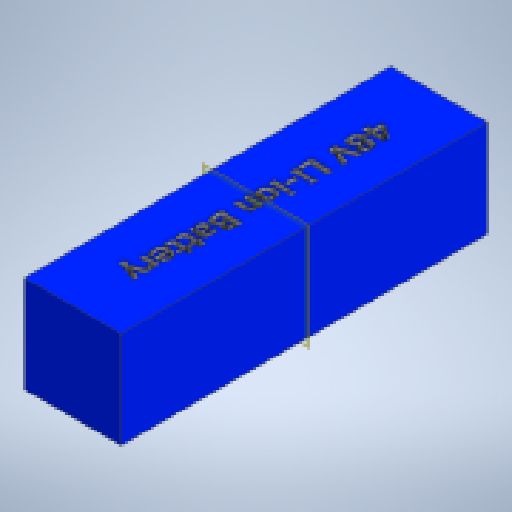
# Autodesk Inventor part: Battery
Saved by Autodesk Inventor 2026.2 (Build 302298010, 298A)
## iProperties
Created: 2026-03-27
Part Number: Battery
Material: Generic
Document SubType Name: Modeling
Designer: chanh
Density: 1 g/cm^3
Appearance: Default
Author: chanh
Autodesk Inventor part; units mm, degrees
ref_plane "YZ Plane" through (0, 0, 0) normal (1, 0, 0) x (0, 1, 0)
ref_plane "XZ Plane" through (0, 0, 0) normal (0, 1, 0) x (-1, 0, 0)
ref_plane "XY Plane" through (0, 0, 0) normal (0, 0, 1) x (1, 0, 0)
sketch "Sketch1" plane through (0, 0, 0) normal (0, 0, 1) x (1, 0, 0)
  line L0 (-35, -35) -> (35, -35)
  line L1 (35, -35) -> (35, 35)
  line L2 (35, 35) -> (-35, 35)
  line L3 (-35, 35) -> (-35, -35)
  line L4 (-35, -35) -> (35, 35) construction
  line L5 (35, -35) -> (-35, 35) construction
  point P0 (0, 0)
  dimension "d0" = 70
  dimension "d1" = 70
  constraints: 12 end point, 2 midpoint, 2 parallel, 1 horizontal, 1 perpendicular
  measures "d0" distance of L1.end L2.end
  measures "d1" distance of L0.end L1.end
extrude "Extrusion1" add sketch "Sketch1" along normal blind 265
sketch "Sketch2" plane through (-35, 35, 0) normal (0, 1, 0) x (1, 0, 0)
  line L0 (44.9615, -38.8119) -> (44.9615, -229.4187) construction
  line L1 (44.9615, -229.4187) -> (21.1166, -229.4187) construction
  line L2 (21.1166, -229.4187) -> (21.1166, -38.8119) construction
  line L3 (21.1166, -38.8119) -> (44.9615, -38.8119) construction
  line L4 (32.7816, -51.5388) -> (32.7816, -49.5088)
  line L5 (32.7816, -49.5088) -> (29.2443, -49.5088)
  line L6 (29.2443, -49.5088) -> (29.2443, -45.8743)
  line L7 (29.2443, -45.8743) -> (32.7816, -45.8743)
  line L8 (32.7816, -45.8743) -> (32.7816, -39.2616)
  line L9 (32.7816, -39.2616) -> (35.5774, -39.2616)
  line L10 (35.5774, -39.2616) -> (44.2808, -45.7527)
  line L11 (44.2808, -45.7527) -> (44.2808, -49.5088)
  line L12 (44.2808, -49.5088) -> (35.4801, -49.5088)
  line L13 (35.4801, -49.5088) -> (35.4801, -51.5388)
  line L14 (35.4801, -51.5388) -> (32.7816, -51.5388)
  line L15 (35.4801, -45.8743) -> (40.5855, -45.8743)
  line L16 (40.5855, -45.8743) -> (35.4801, -42.0696)
  line L17 (35.4801, -42.0696) -> (35.4801, -45.8743)
  spline S0 degree 2 poles (33.4502, -64.4602) (32.4899, -64.4602) (30.8245, -63.6579) (30.2168, -62.8921) knots 0 0 0 1 2 2 2
  spline S1 degree 2 poles (30.2168, -62.8921) (29.609, -62.1263) (28.9283, -59.9261) (28.9283, -58.5039) knots 0 0 0 1 2 2 2
  spline S2 degree 2 poles (28.9283, -58.5039) (28.9283, -56.9845) (29.6211, -54.7114) (30.2168, -53.9821) knots 0 0 0 1 2 2 2
  spline S3 degree 2 poles (30.2168, -53.9821) (30.8124, -53.2649) (32.4291, -52.5842) (33.3286, -52.5842) knots 0 0 0 1 2 2 2
  spline S4 degree 2 poles (33.3286, -52.5842) (34.6171, -52.5842) (36.331, -54.0064) (36.9023, -55.3556) knots 0 0 0 1 2 2 2
  line L18 (36.9023, -55.3556) -> (36.9631, -55.3556)
  spline S5 degree 2 poles (36.9631, -55.3556) (37.6074, -54.0307) (39.4429, -52.9853) (40.5733, -52.9853) knots 0 0 0 1 2 2 2
  spline S6 degree 2 poles (40.5733, -52.9853) (41.3999, -52.9853) (42.8464, -53.7146) (43.4177, -54.4318) knots 0 0 0 1 2 2 2
  spline S7 degree 2 poles (43.4177, -54.4318) (43.9647, -55.1247) (44.6211, -57.2276) (44.6211, -58.5404) knots 0 0 0 1 2 2 2
  spline S8 degree 2 poles (44.6211, -58.5404) (44.6211, -59.9261) (44.0255, -61.9926) (43.5393, -62.6612) knots 0 0 0 1 2 2 2
  spline S9 degree 2 poles (43.5393, -62.6612) (43.0531, -63.3419) (41.643, -64.0712) (40.8286, -64.0712) knots 0 0 0 1 2 2 2
  spline S10 degree 2 poles (40.8286, -64.0712) (39.7589, -64.0712) (38.045, -62.8313) (37.4493, -61.555) knots 0 0 0 1 2 2 2
  line L19 (37.4493, -61.555) -> (37.4007, -61.555)
  spline S11 degree 2 poles (37.4007, -61.555) (36.7929, -63.0501) (34.8237, -64.4602) (33.4502, -64.4602) knots 0 0 0 1 2 2 2
  spline S12 degree 2 poles (33.2921, -60.7406) (34.0336, -60.7406) (34.8116, -60.1085) (35.31, -59.0874) knots 0 0 0 1 2 2 2
  spline S13 degree 2 poles (35.31, -59.0874) (35.4437, -58.7957) (35.8691, -57.6895) (36.0515, -57.2641) knots 0 0 0 1 2 2 2
  spline S14 degree 2 poles (36.0515, -57.2641) (35.6625, -56.8751) (34.4955, -56.2552) (33.8027, -56.2552) knots 0 0 0 1 2 2 2
  spline S15 degree 2 poles (33.8027, -56.2552) (32.7573, -56.2552) (31.5053, -57.5923) (31.5053, -58.6741) knots 0 0 0 1 2 2 2
  spline S16 degree 2 poles (31.5053, -58.6741) (31.5053, -58.978) (31.6997, -59.7317) (31.8942, -60.0234) knots 0 0 0 1 2 2 2
  spline S17 degree 2 poles (31.8942, -60.0234) (32.1252, -60.3516) (32.7573, -60.7406) (33.2921, -60.7406) knots 0 0 0 1 2 2 2
  spline S18 degree 2 poles (40.391, -60.4124) (41.1568, -60.4124) (42.0685, -59.4035) (42.0685, -58.5404) knots 0 0 0 1 2 2 2
  spline S19 degree 2 poles (42.0685, -58.5404) (42.0685, -57.7138) (41.2419, -56.7049) (40.6341, -56.7049) knots 0 0 0 1 2 2 2
  spline S20 degree 2 poles (40.6341, -56.7049) (40.0385, -56.7049) (39.297, -57.3127) (38.9931, -57.9569) knots 0 0 0 1 2 2 2
  spline S21 degree 2 poles (38.9931, -57.9569) (38.8472, -58.2365) (38.5433, -59.0145) (38.3002, -59.6587) knots 0 0 0 1 2 2 2
  spline S22 degree 2 poles (38.3002, -59.6587) (38.8108, -60.0477) (39.7711, -60.4124) (40.391, -60.4124) knots 0 0 0 1 2 2 2
  line L20 (44.2808, -79.1684) -> (29.2808, -74.0145)
  line L21 (29.2808, -74.0145) -> (29.2808, -70.0882)
  line L22 (29.2808, -70.0882) -> (44.2808, -64.9343)
  line L23 (44.2808, -64.9343) -> (44.2808, -68.8362)
  line L24 (44.2808, -68.8362) -> (34.1066, -72.1061)
  line L25 (34.1066, -72.1061) -> (44.2808, -75.3637)
  line L26 (44.2808, -75.3637) -> (44.2808, -79.1684)
  line L27 (29.2808, -96.6117) -> (29.2808, -86.6077)
  line L28 (29.2808, -86.6077) -> (44.2808, -86.6077)
  line L29 (44.2808, -86.6077) -> (44.2808, -90.3759)
  line L30 (44.2808, -90.3759) -> (32.1374, -90.3759)
  line L31 (32.1374, -90.3759) -> (32.1374, -96.6117)
  line L32 (32.1374, -96.6117) -> (29.2808, -96.6117)
  line L33 (29.2808, -101.7292) -> (29.2808, -98.2041)
  line L34 (29.2808, -98.2041) -> (40.5976, -98.2041)
  line L35 (40.5976, -98.2041) -> (40.5976, -101.7292)
  line L36 (40.5976, -101.7292) -> (29.2808, -101.7292)
  line L37 (42.2143, -101.8386) -> (42.2143, -98.1069)
  line L38 (42.2143, -98.1069) -> (44.9615, -98.1069)
  line L39 (44.9615, -98.1069) -> (44.9615, -101.8386)
  line L40 (44.9615, -101.8386) -> (42.2143, -101.8386)
  line L41 (34.5077, -110.8581) -> (34.5077, -104.1847)
  line L42 (34.5077, -104.1847) -> (37.3035, -104.1847)
  line L43 (37.3035, -104.1847) -> (37.3035, -110.8581)
  line L44 (37.3035, -110.8581) -> (34.5077, -110.8581)
  line L45 (29.2808, -116.8508) -> (29.2808, -113.3257)
  line L46 (29.2808, -113.3257) -> (40.5976, -113.3257)
  line L47 (40.5976, -113.3257) -> (40.5976, -116.8508)
  line L48 (40.5976, -116.8508) -> (29.2808, -116.8508)
  line L49 (42.2143, -116.9602) -> (42.2143, -113.2284)
  line L50 (42.2143, -113.2284) -> (44.9615, -113.2284)
  line L51 (44.9615, -113.2284) -> (44.9615, -116.9602)
  line L52 (44.9615, -116.9602) -> (42.2143, -116.9602)
  spline S23 degree 2 poles (34.9331, -130.4043) (32.1374, -130.4043) (28.9283, -127.3532) (28.9283, -124.5696) knots 0 0 0 1 2 2 2
  spline S24 degree 2 poles (28.9283, -124.5696) (28.9283, -121.7981) (32.1374, -118.7227) (34.9331, -118.7227) knots 0 0 0 1 2 2 2
  spline S25 degree 2 poles (34.9331, -118.7227) (37.7532, -118.7227) (40.9502, -121.7981) (40.9502, -124.5696) knots 0 0 0 1 2 2 2
  spline S26 degree 2 poles (40.9502, -124.5696) (40.9502, -127.3411) (37.7411, -130.4043) (34.9331, -130.4043) knots 0 0 0 1 2 2 2
  spline S27 degree 2 poles (34.9088, -126.7941) (35.9177, -126.7941) (37.267, -126.4659) (37.6681, -126.1741) knots 0 0 0 1 2 2 2
  spline S28 degree 2 poles (37.6681, -126.1741) (38.0936, -125.8581) (38.4218, -125.068) (38.4218, -124.5696) knots 0 0 0 1 2 2 2
  spline S29 degree 2 poles (38.4218, -124.5696) (38.4218, -124.0834) (38.1301, -123.3176) (37.7168, -123.0015) knots 0 0 0 1 2 2 2
  spline S30 degree 2 poles (37.7168, -123.0015) (37.3278, -122.6976) (35.9542, -122.333) (34.9088, -122.333) knots 0 0 0 1 2 2 2
  spline S31 degree 2 poles (34.9088, -122.333) (33.8756, -122.333) (32.5993, -122.6733) (32.2103, -122.9529) knots 0 0 0 1 2 2 2
  spline S32 degree 2 poles (32.2103, -122.9529) (31.8213, -123.2325) (31.4566, -124.0834) (31.4566, -124.5939) knots 0 0 0 1 2 2 2
  spline S33 degree 2 poles (31.4566, -124.5939) (31.4566, -125.0193) (31.8213, -125.8945) (32.186, -126.162) knots 0 0 0 1 2 2 2
  spline S34 degree 2 poles (32.186, -126.162) (32.6114, -126.4659) (33.8391, -126.7941) (34.9088, -126.7941) knots 0 0 0 1 2 2 2
  line L53 (29.2808, -142.8637) -> (29.2808, -139.3143)
  line L54 (29.2808, -139.3143) -> (34.8845, -139.3143)
  spline S35 degree 2 poles (34.8845, -139.3143) (35.5774, -139.3143) (36.9388, -139.2049) (37.2549, -139.059) knots 0 0 0 1 2 2 2
  spline S36 degree 2 poles (37.2549, -139.059) (37.6438, -138.8767) (37.972, -138.196) (37.972, -137.6125) knots 0 0 0 1 2 2 2
  spline S37 degree 2 poles (37.972, -137.6125) (37.972, -137.1871) (37.6438, -136.2997) (37.2913, -135.8013) knots 0 0 0 1 2 2 2
  line L55 (37.2913, -135.8013) -> (29.2808, -135.8013)
  line L56 (29.2808, -135.8013) -> (29.2808, -132.2762)
  line L57 (29.2808, -132.2762) -> (40.5976, -132.2762)
  line L58 (40.5976, -132.2762) -> (40.5976, -135.8013)
  line L59 (40.5976, -135.8013) -> (39.3456, -135.8013)
  spline S38 degree 2 poles (39.3456, -135.8013) (40.075, -136.6644) (40.9015, -138.3054) (40.9015, -139.3022) knots 0 0 0 1 2 2 2
  spline S39 degree 2 poles (40.9015, -139.3022) (40.9015, -141.0283) (38.7135, -142.8637) (36.6471, -142.8637) knots 0 0 0 1 2 2 2
  line L60 (36.6471, -142.8637) -> (29.2808, -142.8637)
  spline S40 degree 2 poles (33.8756, -163.7106) (32.7573, -163.7106) (31.0677, -162.8597) (30.5085, -162.1547) knots 0 0 0 1 2 2 2
  spline S41 degree 2 poles (30.5085, -162.1547) (29.8399, -161.3038) (29.2808, -159.286) (29.2808, -157.7179) knots 0 0 0 1 2 2 2
  line L61 (29.2808, -157.7179) -> (29.2808, -151.7252)
  line L62 (29.2808, -151.7252) -> (44.2808, -151.7252)
  line L63 (44.2808, -151.7252) -> (44.2808, -157.0129)
  spline S42 degree 2 poles (44.2808, -157.0129) (44.2808, -158.666) (44.0255, -160.3678) (43.6244, -161.1093) knots 0 0 0 1 2 2 2
  spline S43 degree 2 poles (43.6244, -161.1093) (43.1989, -161.9237) (41.7403, -162.7138) (40.7921, -162.7138) knots 0 0 0 1 2 2 2
  spline S44 degree 2 poles (40.7921, -162.7138) (39.6981, -162.7138) (37.9842, -161.6198) (37.5831, -160.6474) knots 0 0 0 1 2 2 2
  line L64 (37.5831, -160.6474) -> (37.5101, -160.6474)
  spline S45 degree 2 poles (37.5101, -160.6474) (37.2184, -162.0453) (35.4072, -163.7106) (33.8756, -163.7106) knots 0 0 0 1 2 2 2
  spline S46 degree 2 poles (33.9364, -159.8208) (34.6414, -159.8208) (35.4315, -159.2616) (35.6382, -158.7025) knots 0 0 0 1 2 2 2
  spline S47 degree 2 poles (35.6382, -158.7025) (35.7719, -158.3621) (35.7962, -157.1587) (35.7962, -156.162) knots 0 0 0 1 2 2 2
  line L65 (35.7962, -156.162) -> (35.7962, -155.4691)
  line L66 (35.7962, -155.4691) -> (32.0158, -155.4691)
  line L67 (32.0158, -155.4691) -> (32.0158, -155.6757)
  spline S48 degree 2 poles (32.0158, -155.6757) (32.0158, -157.1344) (32.0523, -158.2527) (32.3075, -158.8362) knots 0 0 0 1 2 2 2
  spline S49 degree 2 poles (32.3075, -158.8362) (32.5385, -159.3467) (33.3894, -159.8208) (33.9364, -159.8208) knots 0 0 0 1 2 2 2
  spline S50 degree 2 poles (40.0506, -158.8848) (40.4153, -158.8848) (41.1811, -158.508) (41.3513, -158.119) knots 0 0 0 1 2 2 2
  spline S51 degree 2 poles (41.3513, -158.119) (41.5215, -157.7543) (41.5458, -156.7333) (41.5458, -155.7244) knots 0 0 0 1 2 2 2
  line L68 (41.5458, -155.7244) -> (41.5458, -155.4691)
  line L69 (41.5458, -155.4691) -> (38.361, -155.4691)
  line L70 (38.361, -155.4691) -> (38.361, -155.9432)
  spline S52 degree 2 poles (38.361, -155.9432) (38.361, -156.9035) (38.3975, -157.6814) (38.592, -158.0947) knots 0 0 0 1 2 2 2
  spline S53 degree 2 poles (38.592, -158.0947) (38.8108, -158.5445) (39.5523, -158.8848) (40.0506, -158.8848) knots 0 0 0 1 2 2 2
  spline S54 degree 2 poles (30.4842, -171.9035) (30.1803, -171.5388) (29.6941, -170.9675) (29.451, -170.4813) knots 0 0 0 1 2 2 2
  spline S55 degree 2 poles (29.451, -170.4813) (29.22, -170.0072) (28.9769, -169.1077) (28.9769, -168.3054) knots 0 0 0 1 2 2 2
  spline S56 degree 2 poles (28.9769, -168.3054) (28.9769, -166.7981) (30.9947, -164.8167) (32.5263, -164.8167) knots 0 0 0 1 2 2 2
  spline S57 degree 2 poles (32.5263, -164.8167) (33.7784, -164.8167) (35.3343, -165.8257) (35.784, -166.7738) knots 0 0 0 1 2 2 2
  spline S58 degree 2 poles (35.784, -166.7738) (36.2459, -167.7341) (36.6106, -170.3962) (36.7079, -171.9278) knots 0 0 0 1 2 2 2
  line L71 (36.7079, -171.9278) -> (36.7686, -171.9278)
  spline S59 degree 2 poles (36.7686, -171.9278) (37.7046, -171.9278) (38.4218, -170.542) (38.4218, -169.1563) knots 0 0 0 1 2 2 2
  spline S60 degree 2 poles (38.4218, -169.1563) (38.4218, -168.5364) (37.972, -166.8589) (37.6195, -166.0688) knots 0 0 0 1 2 2 2
  line L72 (37.6195, -166.0688) -> (37.6195, -165.7649)
  line L73 (37.6195, -165.7649) -> (40.3545, -165.7649)
  spline S61 degree 2 poles (40.3545, -165.7649) (40.5004, -166.2876) (40.9137, -168.6214) (40.9137, -169.8127) knots 0 0 0 1 2 2 2
  spline S62 degree 2 poles (40.9137, -169.8127) (40.9137, -172.73) (38.9688, -175.4043) (36.9753, -175.4043) knots 0 0 0 1 2 2 2
  line L74 (36.9753, -175.4043) -> (29.2808, -175.4043)
  line L75 (29.2808, -175.4043) -> (29.2808, -171.9035)
  line L76 (29.2808, -171.9035) -> (30.4842, -171.9035)
  line L77 (32.2346, -171.9035) -> (34.5806, -171.9035)
  spline S63 degree 2 poles (34.5806, -171.9035) (34.4955, -171.0039) (34.3618, -169.8978) (34.1673, -169.3629) knots 0 0 0 1 2 2 2
  spline S64 degree 2 poles (34.1673, -169.3629) (34.0093, -168.8889) (33.3529, -168.3783) (32.8181, -168.3783) knots 0 0 0 1 2 2 2
  spline S65 degree 2 poles (32.8181, -168.3783) (32.0279, -168.3783) (31.4323, -169.2414) (31.4323, -170.0801) knots 0 0 0 1 2 2 2
  spline S66 degree 2 poles (31.4323, -170.0801) (31.4323, -170.542) (31.8578, -171.5145) (32.2346, -171.9035) knots 0 0 0 1 2 2 2
  spline S67 degree 2 poles (29.062, -182.3451) (29.062, -180.1936) (30.8367, -178.2244) (32.8545, -178.2244) knots 0 0 0 1 2 2 2
  line L78 (32.8545, -178.2244) -> (38.1422, -178.2244)
  line L79 (38.1422, -178.2244) -> (38.1422, -176.8751)
  line L80 (38.1422, -176.8751) -> (40.5976, -176.8751)
  line L81 (40.5976, -176.8751) -> (40.5976, -178.2244)
  line L82 (40.5976, -178.2244) -> (43.831, -178.2244)
  line L83 (43.831, -178.2244) -> (43.831, -181.7495)
  line L84 (43.831, -181.7495) -> (40.5976, -181.7495)
  line L85 (40.5976, -181.7495) -> (40.5976, -185.1531)
  line L86 (40.5976, -185.1531) -> (38.1422, -185.1531)
  line L87 (38.1422, -185.1531) -> (38.1422, -181.7495)
  line L88 (38.1422, -181.7495) -> (34.1187, -181.7495)
  spline S68 degree 2 poles (34.1187, -181.7495) (33.5231, -181.7495) (32.6357, -181.7738) (32.2832, -181.9197) knots 0 0 0 1 2 2 2
  spline S69 degree 2 poles (32.2832, -181.9197) (31.9307, -182.0655) (31.5174, -182.7827) (31.5174, -183.4634) knots 0 0 0 1 2 2 2
  spline S70 degree 2 poles (31.5174, -183.4634) (31.5174, -183.7552) (31.7605, -184.6668) (31.8578, -184.8492) knots 0 0 0 1 2 2 2
  line L89 (31.8578, -184.8492) -> (31.8578, -185.1531)
  line L90 (31.8578, -185.1531) -> (29.378, -185.1531)
  spline S71 degree 2 poles (29.378, -185.1531) (29.2322, -184.5817) (29.062, -183.2932) (29.062, -182.3451) knots 0 0 0 1 2 2 2
  spline S72 degree 2 poles (29.062, -190.9148) (29.062, -188.7633) (30.8367, -186.7941) (32.8545, -186.7941) knots 0 0 0 1 2 2 2
  line L91 (32.8545, -186.7941) -> (38.1422, -186.7941)
  line L92 (38.1422, -186.7941) -> (38.1422, -185.4448)
  line L93 (38.1422, -185.4448) -> (40.5976, -185.4448)
  line L94 (40.5976, -185.4448) -> (40.5976, -186.7941)
  line L95 (40.5976, -186.7941) -> (43.831, -186.7941)
  line L96 (43.831, -186.7941) -> (43.831, -190.3192)
  line L97 (43.831, -190.3192) -> (40.5976, -190.3192)
  line L98 (40.5976, -190.3192) -> (40.5976, -193.7227)
  line L99 (40.5976, -193.7227) -> (38.1422, -193.7227)
  line L100 (38.1422, -193.7227) -> (38.1422, -190.3192)
  line L101 (38.1422, -190.3192) -> (34.1187, -190.3192)
  spline S73 degree 2 poles (34.1187, -190.3192) (33.5231, -190.3192) (32.6357, -190.3435) (32.2832, -190.4894) knots 0 0 0 1 2 2 2
  spline S74 degree 2 poles (32.2832, -190.4894) (31.9307, -190.6352) (31.5174, -191.3524) (31.5174, -192.0331) knots 0 0 0 1 2 2 2
  spline S75 degree 2 poles (31.5174, -192.0331) (31.5174, -192.3249) (31.7605, -193.2365) (31.8578, -193.4189) knots 0 0 0 1 2 2 2
  line L102 (31.8578, -193.4189) -> (31.8578, -193.7227)
  line L103 (31.8578, -193.7227) -> (29.378, -193.7227)
  spline S76 degree 2 poles (29.378, -193.7227) (29.2322, -193.1514) (29.062, -191.8629) (29.062, -190.9148) knots 0 0 0 1 2 2 2
  spline S77 degree 2 poles (28.9769, -200.9553) (28.9769, -197.7462) (32.0401, -194.3305) (34.8724, -194.3305) knots 0 0 0 1 2 2 2
  spline S78 degree 2 poles (34.8724, -194.3305) (37.6438, -194.3305) (40.9502, -197.5153) (40.9502, -200.384) knots 0 0 0 1 2 2 2
  spline S79 degree 2 poles (40.9502, -200.384) (40.9502, -202.9731) (38.1422, -205.5988) (35.5409, -205.5988) knots 0 0 0 1 2 2 2
  line L104 (35.5409, -205.5988) -> (34.2646, -205.5988)
  line L105 (34.2646, -205.5988) -> (34.2646, -197.8556)
  spline S80 degree 2 poles (34.2646, -197.8556) (33.4745, -197.9043) (32.4291, -198.4756) (32.113, -198.9375) knots 0 0 0 1 2 2 2
  spline S81 degree 2 poles (32.113, -198.9375) (31.797, -199.3872) (31.5296, -200.6028) (31.5296, -201.32) knots 0 0 0 1 2 2 2
  spline S82 degree 2 poles (31.5296, -201.32) (31.5296, -201.9278) (31.797, -203.119) (32.0279, -203.6174) knots 0 0 0 1 2 2 2
  spline S83 degree 2 poles (32.0279, -203.6174) (32.2103, -204.055) (32.66, -204.7843) (32.8302, -205.0153) knots 0 0 0 1 2 2 2
  line L106 (32.8302, -205.0153) -> (32.8302, -205.3921)
  line L107 (32.8302, -205.3921) -> (29.9129, -205.3921)
  spline S84 degree 2 poles (29.9129, -205.3921) (29.7427, -204.9545) (29.451, -204.2495) (29.3051, -203.6174) knots 0 0 0 1 2 2 2
  spline S85 degree 2 poles (29.3051, -203.6174) (29.1471, -203.0461) (28.9769, -201.8305) (28.9769, -200.9553) knots 0 0 0 1 2 2 2
  spline S86 degree 2 poles (36.3918, -202.1223) (37.5101, -202.0979) (38.6892, -201.1133) (38.6892, -200.1044) knots 0 0 0 1 2 2 2
  spline S87 degree 2 poles (38.6892, -200.1044) (38.6892, -199.0712) (37.4493, -197.9043) (36.3918, -197.8435) knots 0 0 0 1 2 2 2
  line L108 (36.3918, -197.8435) -> (36.3918, -202.1223)
  line L109 (37.2549, -215.0072) -> (37.2549, -214.7155)
  spline S88 degree 2 poles (37.2549, -214.7155) (37.3278, -214.5088) (37.4007, -213.743) (37.4007, -213.2811) knots 0 0 0 1 2 2 2
  spline S89 degree 2 poles (37.4007, -213.2811) (37.4007, -212.7341) (37.0725, -211.5064) (36.8537, -210.9351) knots 0 0 0 1 2 2 2
  line L110 (36.8537, -210.9351) -> (29.2808, -210.9351)
  line L111 (29.2808, -210.9351) -> (29.2808, -207.4099)
  line L112 (29.2808, -207.4099) -> (40.5976, -207.4099)
  line L113 (40.5976, -207.4099) -> (40.5976, -210.9351)
  line L114 (40.5976, -210.9351) -> (38.9688, -210.9351)
  spline S90 degree 2 poles (38.9688, -210.9351) (39.1876, -211.1782) (39.8683, -212.0291) (40.075, -212.3816) knots 0 0 0 1 2 2 2
  spline S91 degree 2 poles (40.075, -212.3816) (40.3059, -212.7706) (40.6341, -213.7916) (40.6341, -214.2414) knots 0 0 0 1 2 2 2
  spline S92 degree 2 poles (40.6341, -214.2414) (40.6341, -214.4116) (40.6098, -214.837) (40.5976, -215.0072) knots 0 0 0 1 2 2 2
  line L115 (40.5976, -215.0072) -> (37.2549, -215.0072)
  line L116 (40.5976, -226.9075) -> (25.1357, -221.2065)
  line L117 (25.1357, -221.2065) -> (25.1357, -217.414)
  line L118 (25.1357, -217.414) -> (29.5604, -219.1279)
  line L119 (29.5604, -219.1279) -> (40.5976, -214.9829)
  line L120 (40.5976, -214.9829) -> (40.5976, -218.6782)
  line L121 (40.5976, -218.6782) -> (33.4988, -221.0607)
  line L122 (33.4988, -221.0607) -> (40.5976, -223.2851)
  line L123 (40.5976, -223.2851) -> (40.5976, -226.9075)
  point P0 (35, 0)
  constraints: 2 other
extrude "Extrusion2" cut sketch "Sketch2" against normal blind 10
ref_plane "Work Plane1" through (0, 0, 132.5) normal (0, 0, -1) x (-1, 0, 0)
body "Solid1"
